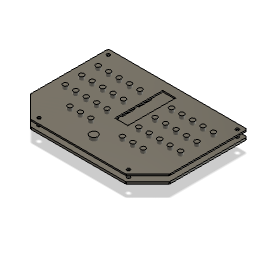
HandyPi_Keyboard (Autodesk Fusion 360 design; units mm, degrees)
Autodesk Fusion 360 part; units mm, degrees
(part 1 of 2)
sketch "basePCB" plane through (0, 0, 0) normal (0, 1, 0) x (1, 0, 0)
  line L0 (-37.295, 35.389) -> (-37.295, 28.289)
  circle A0 centre (-43.588, 31.486) radius 2.25
  line L1 (-37.295, 28.289) -> (-34.895, 28.289)
  line L2 (-0.936, -12.156) -> (-3.436, -12.156)
  line L3 (-28.672, 28.162) -> (-28.672, 35.262)
  line L4 (1.39, -12.156) -> (1.39, -16.756)
  line L5 (3.89, -12.156) -> (1.39, -12.156)
  line L6 (-0.936, -16.756) -> (-0.936, -12.156)
  line L7 (-3.436, -12.156) -> (-3.436, -16.756)
  line L8 (1.39, -16.756) -> (3.89, -16.756)
  line L9 (-3.436, -16.756) -> (-0.936, -16.756)
  line L10 (3.89, -16.756) -> (3.89, -12.156)
  line L11 (-34.895, 35.389) -> (-37.295, 35.389)
  line L12 (-31.072, 28.162) -> (-28.672, 28.162)
  line L13 (-28.672, 35.262) -> (-31.072, 35.262)
  line L14 (-31.072, 35.262) -> (-31.072, 28.162)
  line L15 (-34.895, 28.289) -> (-34.895, 35.389)
  line L16 (-15.998, -11.806) -> (-15.998, -11.556)
  line L17 (-8.124, 25.528) -> (-8.374, 25.528)
  line L18 (31.5, 25.528) -> (31.25, 25.528)
  line L19 (23.626, -11.556) -> (23.376, -11.556)
  line L20 (31.572, 3.582) -> (31.572, 3.832)
  line L21 (31.5, 25.278) -> (31.5, 16.278)
  line L22 (8.252, -11.806) -> (8.252, -11.556)
  line L23 (-8.124, -11.806) -> (-8.124, -11.556)
  line L24 (31.5, -11.806) -> (31.5, -20.806)
  line L25 (23.626, 16.028) -> (23.626, 16.278)
  line L26 (-23.498, 25.528) -> (-23.248, 25.528)
  line L27 (16.126, 25.528) -> (16.376, 25.528)
  line L28 (-8.374, -8.76) -> (-8.124, -8.76)
  line L29 (-15.624, 0.49) -> (-15.624, 0.74)
  line L30 (23.376, -21.056) -> (23.626, -21.056)
  line L31 (-15.624, 16.028) -> (-15.624, 16.278)
  line L32 (-8.124, 16.028) -> (-8.124, 16.278)
  line L33 (15.752, -11.556) -> (15.502, -11.556)
  line L34 (8.252, 13.082) -> (8.502, 13.082)
  line L35 (24.25, 0.74) -> (31.25, 0.74)
  line L36 (15.752, 25.278) -> (15.752, 25.528)
  line L37 (-15.998, -8.76) -> (-15.998, -8.51)
  line L38 (-15.624, 16.278) -> (-15.624, 25.278)
  line L39 (24, 16.028) -> (24, 16.278)
  line L40 (8.252, 25.528) -> (8.502, 25.528)
  line L41 (15.752, -8.76) -> (15.752, -8.51)
  line L42 (31.5, 0.49) -> (31.5, -8.51)
  line L43 (8.252, 0.49) -> (8.252, 0.74)
  line L44 (16.126, -8.51) -> (16.126, 0.49)
  line L45 (15.752, -11.806) -> (15.752, -20.806)
  line L46 (8.502, 13.082) -> (15.502, 13.082)
  line L47 (23.626, -21.056) -> (23.626, -20.806)
  line L48 (15.752, 13.082) -> (15.502, 13.082)
  line L49 (16.376, -21.056) -> (16.126, -21.056)
  line L50 (16.126, 0.49) -> (16.126, 0.74)
  line L51 (31.874, -8.51) -> (31.874, 0.49)
  line L52 (23.626, 0.49) -> (23.626, -8.51)
  line L53 (-15.624, -11.556) -> (-15.374, -11.556)
  line L54 (16.376, 25.528) -> (23.376, 25.528)
  line L55 (31.5, 0.49) -> (31.5, 0.74)
  line L56 (31.5, -8.76) -> (31.5, -8.51)
  line L57 (31.874, 25.278) -> (31.874, 25.528)
  line L58 (-16.248, -8.76) -> (-15.998, -8.76)
  line L59 (24, -11.556) -> (24.25, -11.556)
  line L60 (8.502, 3.582) -> (8.252, 3.582)
  line L61 (31.5, -11.556) -> (31.25, -11.556)
  line L62 (39.374, -8.76) -> (39.374, -8.51)
  line L63 (31.322, 3.582) -> (24.322, 3.582)
  line L64 (16.126, -8.76) -> (16.126, -8.51)
  line L65 (-23.498, -8.51) -> (-23.498, 0.49)
  line L66 (16.126, 12.832) -> (16.126, 13.082)
  line L67 (24, 16.278) -> (24, 25.278)
  line L68 (15.502, -8.76) -> (15.752, -8.76)
  line L69 (24.25, -21.056) -> (24, -21.056)
  line L70 (23.626, 12.832) -> (23.626, 13.082)
  line L71 (-8.374, -21.056) -> (-8.124, -21.056)
  line L72 (-8.374, 16.028) -> (-15.374, 16.028)
  line L73 (24.25, 16.028) -> (24, 16.028)
  line L74 (16.126, -11.806) -> (16.126, -11.556)
  line L75 (-15.624, -20.806) -> (-15.624, -11.806)
  line L76 (15.752, -11.806) -> (15.752, -11.556)
  line L77 (-15.998, 0.74) -> (-16.248, 0.74)
  line L78 (24.322, 13.082) -> (31.322, 13.082)
  line L79 (-15.998, -11.806) -> (-15.998, -20.806)
  line L80 (31.322, 3.582) -> (31.572, 3.582)
  line L81 (16.126, 16.028) -> (16.126, 16.278)
  line L82 (39.124, -8.76) -> (39.374, -8.76)
  line L83 (-8.124, -21.056) -> (-8.124, -20.806)
  line L84 (23.626, 25.278) -> (23.626, 25.528)
  line L85 (23.626, 13.082) -> (23.376, 13.082)
  line L86 (-15.374, 0.74) -> (-8.374, 0.74)
  line L87 (8.502, -8.76) -> (8.252, -8.76)
  line L88 (39.124, 16.028) -> (39.374, 16.028)
  line L89 (-8.124, -11.556) -> (-8.374, -11.556)
  line L90 (31.572, 13.082) -> (31.322, 13.082)
  line L91 (31.5, 16.028) -> (31.5, 16.278)
  line L92 (-16.248, -21.056) -> (-15.998, -21.056)
  line L93 (-15.624, 25.278) -> (-15.624, 25.528)
  line L94 (32.196, 3.582) -> (31.946, 3.582)
  line L95 (39.374, 25.528) -> (39.124, 25.528)
  line L96 (8.252, -11.556) -> (8.502, -11.556)
  line L97 (16.376, 13.082) -> (23.376, 13.082)
  line L98 (31.5, -11.806) -> (31.5, -11.556)
  line L99 (8.502, 16.028) -> (8.252, 16.028)
  line L100 (15.502, 3.582) -> (15.752, 3.582)
  line L101 (24.072, 12.832) -> (24.072, 13.082)
  line L102 (-23.498, 25.278) -> (-23.498, 25.528)
  line L103 (8.252, 25.278) -> (8.252, 25.528)
  line L104 (-15.374, -21.056) -> (-15.624, -21.056)
  line L105 (15.502, 3.582) -> (8.502, 3.582)
  line L106 (-23.498, 0.74) -> (-23.248, 0.74)
  line L107 (8.502, -21.056) -> (8.252, -21.056)
  line L108 (16.126, -21.056) -> (16.126, -20.806)
  line L109 (31.25, -21.056) -> (31.5, -21.056)
  line L110 (8.502, 0.74) -> (15.502, 0.74)
  line L111 (39.446, 3.582) -> (39.446, 3.832)
  line L112 (39.196, 3.582) -> (39.446, 3.582)
  line L113 (-23.248, 0.74) -> (-16.248, 0.74)
  line L114 (15.752, 3.582) -> (15.752, 3.832)
  line L115 (15.502, -8.76) -> (8.502, -8.76)
  line L116 (39.446, 12.832) -> (39.446, 13.082)
  line L117 (-15.624, -11.806) -> (-15.624, -11.556)
  line L118 (39.374, 25.278) -> (39.374, 25.528)
  line L119 (-15.374, -11.556) -> (-8.374, -11.556)
  line L120 (-15.998, -21.056) -> (-15.998, -20.806)
  line L121 (16.376, -8.76) -> (16.126, -8.76)
  line L122 (-15.624, 25.528) -> (-15.374, 25.528)
  line L123 (31.5, 25.278) -> (31.5, 25.528)
  line L124 (15.752, 12.832) -> (15.752, 3.832)
  line L125 (16.376, 0.74) -> (23.376, 0.74)
  line L126 (-16.248, -21.056) -> (-23.248, -21.056)
  line L127 (16.376, 3.582) -> (16.126, 3.582)
  line L128 (23.376, 16.028) -> (16.376, 16.028)
  line L129 (-23.248, -8.76) -> (-23.498, -8.76)
  line L130 (16.376, -11.556) -> (23.376, -11.556)
  line L131 (24, 0.74) -> (24.25, 0.74)
  line L132 (-23.498, -8.76) -> (-23.498, -8.51)
  line L133 (-23.498, -11.556) -> (-23.248, -11.556)
  line L134 (23.376, -8.76) -> (23.626, -8.76)
  line L135 (32.124, 25.528) -> (39.124, 25.528)
  line L136 (31.874, 25.528) -> (32.124, 25.528)
  line L137 (8.252, -21.056) -> (8.252, -20.806)
  line L138 (16.126, 13.082) -> (16.376, 13.082)
  line L139 (32.124, -8.76) -> (31.874, -8.76)
  line L140 (39.124, 16.028) -> (32.124, 16.028)
  line L141 (39.374, 16.028) -> (39.374, 16.278)
  line L142 (24, 0.49) -> (24, 0.74)
  line L143 (23.626, 12.832) -> (23.626, 3.832)
  line L144 (-15.998, 0.49) -> (-15.998, 0.74)
  line L145 (-16.248, -8.76) -> (-23.248, -8.76)
  line L146 (31.25, 16.028) -> (24.25, 16.028)
  line L147 (31.946, 3.582) -> (31.946, 3.832)
  line L148 (31.874, 16.278) -> (31.874, 25.278)
  line L149 (31.25, 16.028) -> (31.5, 16.028)
  line L150 (39.196, 3.582) -> (32.196, 3.582)
  line L151 (16.376, 16.028) -> (16.126, 16.028)
  line L152 (-8.374, -8.76) -> (-15.374, -8.76)
  line L153 (31.25, -8.76) -> (31.5, -8.76)
  line L154 (16.126, 0.74) -> (16.376, 0.74)
  line L155 (8.252, 3.582) -> (8.252, 3.832)
  line L156 (24.072, 3.582) -> (24.072, 3.832)
  line L157 (23.376, 3.582) -> (23.626, 3.582)
  line L158 (16.126, 3.832) -> (16.126, 12.832)
  line L159 (8.252, 16.028) -> (8.252, 16.278)
  line L160 (15.752, -21.056) -> (15.752, -20.806)
  line L161 (8.252, 16.278) -> (8.252, 25.278)
  line L162 (31.946, 3.832) -> (31.946, 12.832)
  line L163 (23.626, 0.74) -> (23.376, 0.74)
  line L164 (24.072, 13.082) -> (24.322, 13.082)
  line L165 (-15.624, -21.056) -> (-15.624, -20.806)
  line L166 (24.322, 3.582) -> (24.072, 3.582)
  line L167 (31.874, 16.028) -> (31.874, 16.278)
  line L168 (39.446, 13.082) -> (39.196, 13.082)
  line L169 (-8.374, 16.028) -> (-8.124, 16.028)
  line L170 (-8.124, 0.74) -> (-8.374, 0.74)
  line L171 (24, -11.806) -> (24, -11.556)
  line L172 (-15.374, 25.528) -> (-8.374, 25.528)
  line L173 (-8.124, -11.806) -> (-8.124, -20.806)
  line L174 (31.946, 12.832) -> (31.946, 13.082)
  line L175 (16.126, 25.278) -> (16.126, 25.528)
  line L176 (23.626, -8.76) -> (23.626, -8.51)
  line L177 (23.376, -8.76) -> (16.376, -8.76)
  line L178 (-8.124, -8.76) -> (-8.124, -8.51)
  line L179 (-15.374, -8.76) -> (-15.624, -8.76)
  line L180 (8.252, 0.74) -> (8.502, 0.74)
  line L181 (16.126, 3.582) -> (16.126, 3.832)
  line L182 (39.124, -8.76) -> (32.124, -8.76)
  line L183 (15.752, 0.49) -> (15.752, -8.51)
  line L184 (-15.374, 16.028) -> (-15.624, 16.028)
  line L185 (-15.998, 25.278) -> (-15.998, 25.528)
  line L186 (16.126, -20.806) -> (16.126, -11.806)
  line L187 (8.252, -8.76) -> (8.252, -8.51)
  line L188 (15.752, 16.028) -> (15.752, 16.278)
  line L189 (15.752, 0.74) -> (15.502, 0.74)
  line L190 (23.626, 25.528) -> (23.376, 25.528)
  line L191 (8.252, -20.806) -> (8.252, -11.806)
  line L192 (15.502, 16.028) -> (8.502, 16.028)
  line L193 (-15.624, -8.51) -> (-15.624, 0.49)
  line L194 (-23.248, -21.056) -> (-23.498, -21.056)
  line L195 (31.572, 12.832) -> (31.572, 13.082)
  line L196 (31.25, -8.76) -> (24.25, -8.76)
  line L197 (15.752, 0.49) -> (15.752, 0.74)
  line L198 (39.374, 0.49) -> (39.374, -8.51)
  line L199 (32.196, 13.082) -> (39.196, 13.082)
  line L200 (-23.498, 0.49) -> (-23.498, 0.74)
  line L201 (32.124, 0.74) -> (39.124, 0.74)
  line L202 (8.502, -11.556) -> (15.502, -11.556)
  line L203 (31.5, -21.056) -> (31.5, -20.806)
  line L204 (16.126, 16.278) -> (16.126, 25.278)
  line L205 (-15.998, -11.556) -> (-16.248, -11.556)
  line L206 (15.502, 16.028) -> (15.752, 16.028)
  line L207 (8.252, -8.51) -> (8.252, 0.49)
  line L208 (-8.124, 25.278) -> (-8.124, 16.278)
  line L209 (24, -21.056) -> (24, -20.806)
  line L210 (-23.498, -20.806) -> (-23.498, -11.806)
  line L211 (-8.124, 25.278) -> (-8.124, 25.528)
  line L212 (23.626, -11.806) -> (23.626, -11.556)
  line L213 (-15.998, 0.49) -> (-15.998, -8.51)
  line L214 (24, -8.51) -> (24, 0.49)
  line L215 (-8.124, 0.49) -> (-8.124, 0.74)
  line L216 (23.376, -21.056) -> (16.376, -21.056)
  line L217 (24, -20.806) -> (24, -11.806)
  line L218 (31.25, -21.056) -> (24.25, -21.056)
  line L219 (31.572, 12.832) -> (31.572, 3.832)
  line L220 (31.874, -8.76) -> (31.874, -8.51)
  line L221 (24.072, 3.832) -> (24.072, 12.832)
  line L222 (15.502, -21.056) -> (15.752, -21.056)
  line L223 (23.626, 3.582) -> (23.626, 3.832)
  line L224 (-8.374, -21.056) -> (-15.374, -21.056)
  line L225 (23.626, 0.49) -> (23.626, 0.74)
  line L226 (-23.248, -11.556) -> (-16.248, -11.556)
  line L227 (-15.624, -8.76) -> (-15.624, -8.51)
  line L228 (15.502, -21.056) -> (8.502, -21.056)
  line L229 (15.752, 25.278) -> (15.752, 16.278)
  line L230 (24.25, -11.556) -> (31.25, -11.556)
  line L231 (8.252, 3.832) -> (8.252, 12.832)
  line L232 (23.376, 3.582) -> (16.376, 3.582)
  line L233 (23.626, 25.278) -> (23.626, 16.278)
  line L234 (31.946, 13.082) -> (32.196, 13.082)
  line L235 (23.626, -11.806) -> (23.626, -20.806)
  line L236 (24, 25.528) -> (24.25, 25.528)
  line L237 (15.752, 12.832) -> (15.752, 13.082)
  line L238 (15.752, 25.528) -> (15.502, 25.528)
  line L239 (8.502, 25.528) -> (15.502, 25.528)
  line L240 (-23.498, -21.056) -> (-23.498, -20.806)
  line L241 (39.374, 25.278) -> (39.374, 16.278)
  line L242 (32.124, 16.028) -> (31.874, 16.028)
  line L243 (24, -8.76) -> (24, -8.51)
  line L244 (23.376, 16.028) -> (23.626, 16.028)
  line L245 (39.446, 12.832) -> (39.446, 3.832)
  line L246 (-15.998, 25.528) -> (-16.248, 25.528)
  line L247 (16.126, -11.556) -> (16.376, -11.556)
  line L248 (31.5, 0.74) -> (31.25, 0.74)
  line L249 (-8.124, 0.49) -> (-8.124, -8.51)
  line L250 (24.25, 25.528) -> (31.25, 25.528)
  line L251 (24.25, -8.76) -> (24, -8.76)
  line L252 (-15.624, 0.74) -> (-15.374, 0.74)
  line L253 (24, 25.278) -> (24, 25.528)
  line L254 (-23.498, -11.806) -> (-23.498, -11.556)
  line L255 (8.252, 12.832) -> (8.252, 13.082)
  line L256 (-31.746, 3.582) -> (-31.746, 3.832)
  line L257 (-47.12, 3.582) -> (-47.12, 3.832)
  line L258 (44.166, 32.996) -> (44.166, 36.096)
  line L259 (-39.87, -8.76) -> (-46.87, -8.76)
  line L260 (-23.872, 25.278) -> (-23.872, 16.278)
  line L261 (-39.246, 3.582) -> (-39.246, 3.832)
  line L262 (-38.996, -8.76) -> (-39.246, -8.76)
  line L263 (-31.746, 0.74) -> (-31.996, 0.74)
  line L264 (-39.87, 3.582) -> (-46.87, 3.582)
  line L265 (16.322, 32.03) -> (28.582, 32.03)
  line L266 (-47.12, 16.028) -> (-47.12, 16.278)
  line L267 (44.166, 36.096) -> (38.066, 36.096)
  line L268 (-31.372, 3.582) -> (-31.372, 3.832)
  line L269 (47.124, 28.22) -> (47.124, 31.22)
  line L270 (-23.872, 25.528) -> (-24.122, 25.528)
  line L271 (-24.122, 16.028) -> (-31.122, 16.028)
  line L272 (-23.872, 0.49) -> (-23.872, 0.74)
  line L273 (-31.372, -11.556) -> (-31.122, -11.556)
  line L274 (-31.746, 12.832) -> (-31.746, 13.082)
  line L275 (-23.872, -11.556) -> (-24.122, -11.556)
  line L276 (-31.372, 13.082) -> (-31.122, 13.082)
  line L277 (-24.122, 3.582) -> (-23.872, 3.582)
  line L278 (-39.62, -8.76) -> (-39.62, -8.51)
  line L279 (-47.12, 25.528) -> (-46.87, 25.528)
  line L280 (-46.87, 25.528) -> (-39.87, 25.528)
  line L281 (-24.122, -8.76) -> (-23.872, -8.76)
  line L282 (-39.246, 16.028) -> (-39.246, 16.278)
  line L283 (-47.12, 0.49) -> (-47.12, 0.74)
  line L284 (-46.87, 3.582) -> (-47.12, 3.582)
  line L285 (-31.746, 0.49) -> (-31.746, 0.74)
  line L286 (-31.372, -21.056) -> (-31.372, -20.806)
  line L287 (-31.122, 25.528) -> (-24.122, 25.528)
  line L288 (-31.746, 16.028) -> (-31.746, 16.278)
  line L289 (-16.248, 16.028) -> (-23.248, 16.028)
  line L290 (-39.62, 25.278) -> (-39.62, 25.528)
  line L291 (-31.746, 13.082) -> (-31.996, 13.082)
  line L292 (-23.872, 0.74) -> (-24.122, 0.74)
  line L293 (-23.872, -8.76) -> (-23.872, -8.51)
  line L294 (-47.12, 3.832) -> (-47.12, 12.832)
  line L295 (38.066, 36.096) -> (38.066, 32.996)
  line L296 (-31.122, 0.74) -> (-24.122, 0.74)
  line L297 (16.068, 28.22) -> (28.328, 28.22)
  line L298 (-24.122, -21.056) -> (-23.872, -21.056)
  line L299 (34.864, 31.22) -> (34.864, 28.22)
  line L300 (-23.248, 16.028) -> (-23.498, 16.028)
  line L301 (-31.996, -8.76) -> (-38.996, -8.76)
  line L302 (-31.996, 16.028) -> (-31.746, 16.028)
  line L303 (-39.246, 25.528) -> (-38.996, 25.528)
  line L304 (-39.87, 3.582) -> (-39.62, 3.582)
  line L305 (28.328, 28.22) -> (28.328, 31.22)
  line L306 (-24.122, -21.056) -> (-31.122, -21.056)
  line L307 (-31.746, 25.278) -> (-31.746, 25.528)
  line L308 (-39.246, 0.49) -> (-39.246, 0.74)
  line L309 (-38.996, 13.082) -> (-31.996, 13.082)
  line L310 (-47.12, -8.51) -> (-47.12, 0.49)
  line L311 (-23.872, -11.806) -> (-23.872, -11.556)
  line L312 (-39.62, 13.082) -> (-39.87, 13.082)
  line L313 (-31.996, -8.76) -> (-31.746, -8.76)
  line L314 (-31.372, 0.49) -> (-31.372, 0.74)
  line L315 (-31.372, 25.528) -> (-31.122, 25.528)
  line L316 (-39.87, 16.028) -> (-39.62, 16.028)
  line L317 (16.322, 35.03) -> (16.322, 32.03)
  line L318 (-31.122, -21.056) -> (-31.372, -21.056)
  line L319 (-16.248, 16.028) -> (-15.998, 16.028)
  line L320 (-23.872, 12.832) -> (-23.872, 3.832)
  line L321 (-31.746, 25.528) -> (-31.996, 25.528)
  line L322 (28.582, 32.03) -> (28.582, 35.03)
  line L323 (-46.87, 13.082) -> (-39.87, 13.082)
  line L324 (-23.248, 25.528) -> (-16.248, 25.528)
  line L325 (-23.872, 3.582) -> (-23.872, 3.832)
  line L326 (-31.372, -8.51) -> (-31.372, 0.49)
  line L327 (-31.996, 16.028) -> (-38.996, 16.028)
  line L328 (-39.62, 12.832) -> (-39.62, 13.082)
  line L329 (-39.246, 3.832) -> (-39.246, 12.832)
  line L330 (-39.62, 3.582) -> (-39.62, 3.832)
  line L331 (-23.498, 16.278) -> (-23.498, 25.278)
  line L332 (-31.122, -8.76) -> (-31.372, -8.76)
  line L333 (-31.746, 25.278) -> (-31.746, 16.278)
  line L334 (-31.996, 3.582) -> (-31.746, 3.582)
  line L335 (-39.87, 16.028) -> (-46.87, 16.028)
  line L336 (-46.87, -8.76) -> (-47.12, -8.76)
  line L337 (38.066, 32.996) -> (44.166, 32.996)
  line L338 (-23.302, 28.22) -> (-11.042, 28.22)
  line L339 (-31.372, 0.74) -> (-31.122, 0.74)
  line L340 (-31.372, 25.278) -> (-31.372, 25.528)
  line L341 (-46.87, 0.74) -> (-39.87, 0.74)
  line L342 (-31.372, -11.806) -> (-31.372, -11.556)
  line L343 (-39.246, 0.74) -> (-38.996, 0.74)
  line L344 (-46.87, 16.028) -> (-47.12, 16.028)
  line L345 (-31.372, 16.028) -> (-31.372, 16.278)
  line L346 (-39.62, 0.49) -> (-39.62, -8.51)
  line L347 (-31.996, 3.582) -> (-38.996, 3.582)
  line L348 (-47.12, 16.278) -> (-47.12, 25.278)
  line L349 (-31.372, -8.76) -> (-31.372, -8.51)
  line L350 (28.328, 31.22) -> (16.068, 31.22)
  line L351 (-39.62, 16.028) -> (-39.62, 16.278)
  line L352 (-24.122, 3.582) -> (-31.122, 3.582)
  line L353 (-11.042, 28.22) -> (-11.042, 31.22)
  line L354 (-23.872, 0.49) -> (-23.872, -8.51)
  line L355 (-31.372, -20.806) -> (-31.372, -11.806)
  line L356 (-23.872, 12.832) -> (-23.872, 13.082)
  line L357 (-23.872, 25.278) -> (-23.872, 25.528)
  line L358 (34.864, 28.22) -> (47.124, 28.22)
  line L359 (-31.746, 0.49) -> (-31.746, -8.51)
  line L360 (-47.12, 0.74) -> (-46.87, 0.74)
  line L361 (-39.62, 0.49) -> (-39.62, 0.74)
  line L362 (-24.122, 16.028) -> (-23.872, 16.028)
  line L363 (-39.62, 12.832) -> (-39.62, 3.832)
  line L364 (-15.998, 16.028) -> (-15.998, 16.278)
  line L365 (-38.996, 3.582) -> (-39.246, 3.582)
  line L366 (-47.12, 25.278) -> (-47.12, 25.528)
  line L367 (-23.872, 13.082) -> (-24.122, 13.082)
  line L368 (-39.246, -8.76) -> (-39.246, -8.51)
  line L369 (47.124, 31.22) -> (34.864, 31.22)
  line L370 (-38.996, 16.028) -> (-39.246, 16.028)
  line L371 (-39.246, -8.51) -> (-39.246, 0.49)
  line L372 (-31.122, -11.556) -> (-24.122, -11.556)
  line L373 (-39.87, -8.76) -> (-39.62, -8.76)
  line L374 (28.582, 35.03) -> (16.322, 35.03)
  line L375 (-39.62, 25.278) -> (-39.62, 16.278)
  line L376 (-39.62, 25.528) -> (-39.87, 25.528)
  line L377 (-24.122, -8.76) -> (-31.122, -8.76)
  line L378 (-23.872, 16.028) -> (-23.872, 16.278)
  line L379 (-31.746, -8.76) -> (-31.746, -8.51)
  line L380 (-39.62, 0.74) -> (-39.87, 0.74)
  line L381 (-47.12, -8.76) -> (-47.12, -8.51)
  line L382 (-31.122, 16.028) -> (-31.372, 16.028)
  line L383 (-31.122, 3.582) -> (-31.372, 3.582)
  line L384 (-23.302, 31.22) -> (-23.302, 28.22)
  line L385 (16.068, 31.22) -> (16.068, 28.22)
  line L386 (-39.246, 12.832) -> (-39.246, 13.082)
  line L387 (-39.246, 13.082) -> (-38.996, 13.082)
  line L388 (-38.996, 25.528) -> (-31.996, 25.528)
  line L389 (-47.12, 13.082) -> (-46.87, 13.082)
  line L390 (-31.372, 3.832) -> (-31.372, 12.832)
  line L391 (-23.872, -21.056) -> (-23.872, -20.806)
  line L392 (-31.372, 16.278) -> (-31.372, 25.278)
  line L393 (-47.12, 12.832) -> (-47.12, 13.082)
  line L394 (-31.372, 12.832) -> (-31.372, 13.082)
  line L395 (-39.246, 16.278) -> (-39.246, 25.278)
  line L396 (-38.996, 0.74) -> (-31.996, 0.74)
  line L397 (-23.872, -11.806) -> (-23.872, -20.806)
  line L398 (-15.998, 25.278) -> (-15.998, 16.278)
  line L399 (-11.042, 31.22) -> (-23.302, 31.22)
  line L400 (-31.122, 13.082) -> (-24.122, 13.082)
  line L401 (-31.746, 12.832) -> (-31.746, 3.832)
  line L402 (-39.246, 25.278) -> (-39.246, 25.528)
  line L403 (-23.498, 16.028) -> (-23.498, 16.278)
  line L404 (46.998, 16.028) -> (39.998, 16.028)
  line L405 (4.99, 31.016) -> (-4.81, 31.016)
  line L406 (47.248, 16.028) -> (47.248, 16.278)
  line L407 (-15.998, 3.582) -> (-15.998, 3.832)
  line L408 (46.998, -8.76) -> (39.998, -8.76)
  line L409 (39.998, 3.582) -> (39.748, 3.582)
  line L410 (-11.958, 35.334) -> (-15.558, 35.334)
  line L411 (-23.248, 13.082) -> (-16.248, 13.082)
  line L412 (-8.124, 12.832) -> (-8.124, 13.082)
  line L413 (46.998, 16.028) -> (47.248, 16.028)
  line L414 (-8.124, 12.832) -> (-8.124, 3.832)
  line L415 (-19.07, 32.234) -> (-19.07, 35.334)
  line L416 (39.748, -8.51) -> (39.748, 0.49)
  line L417 (-8.124, 13.082) -> (-8.374, 13.082)
  line L418 (4.99, -5.084) -> (4.99, 31.016)
  line L419 (39.748, 16.278) -> (39.748, 25.278)
  line L420 (39.374, 0.49) -> (39.374, 0.74)
  line L421 (39.748, -8.76) -> (39.748, -8.51)
  line L422 (-51.208, 37.594) -> (51.154, 37.594)
  arc A1 (-51.208, 37.594) -> (-52.478, 36.324) centre (-51.208, 36.324) ccw
  line L423 (-15.624, 3.582) -> (-15.624, 3.832)
  line L424 (-4.81, 31.016) -> (-4.81, -5.084)
  line L425 (-16.248, 3.582) -> (-23.248, 3.582)
  line L426 (-15.374, 3.582) -> (-15.624, 3.582)
  line L427 (39.748, 12.832) -> (39.748, 13.082)
  line L428 (39.998, 16.028) -> (39.748, 16.028)
  circle A2 centre (48.614, -33.78) radius 2.45
  line L429 (46.998, 3.582) -> (39.998, 3.582)
  line L430 (51.154, -37.59) -> (-51.208, -37.59)
  line L431 (-8.374, 3.582) -> (-8.124, 3.582)
  circle A3 centre (-48.668, -33.78) radius 2.45
  line L432 (39.748, 3.582) -> (39.748, 3.832)
  line L433 (-15.998, 13.082) -> (-16.248, 13.082)
  line L434 (-23.498, 12.832) -> (-23.498, 13.082)
  line L435 (39.748, 13.082) -> (39.998, 13.082)
  line L436 (47.248, 25.528) -> (46.998, 25.528)
  line L437 (-15.374, 13.082) -> (-8.374, 13.082)
  line L438 (39.998, 13.082) -> (46.998, 13.082)
  line L439 (39.998, -8.76) -> (39.748, -8.76)
  arc A4 (52.424, 36.324) -> (51.154, 37.594) centre (51.154, 36.324) ccw
  line L440 (31.874, 0.74) -> (32.124, 0.74)
  line L441 (39.374, 0.74) -> (39.124, 0.74)
  line L442 (39.748, 25.278) -> (39.748, 25.528)
  line L443 (47.248, 0.74) -> (46.998, 0.74)
  line L444 (6.14, -11.688) -> (6.14, -6.088)
  line L445 (39.748, 3.832) -> (39.748, 12.832)
  line L446 (-5.76, -11.688) -> (6.14, -11.688)
  line L447 (39.748, 0.49) -> (39.748, 0.74)
  line L448 (-16.248, 3.582) -> (-15.998, 3.582)
  line L449 (39.998, 25.528) -> (46.998, 25.528)
  line L450 (-23.248, 3.582) -> (-23.498, 3.582)
  line L451 (-8.124, 3.582) -> (-8.124, 3.832)
  line L452 (-15.558, 35.334) -> (-15.558, 32.234)
  line L453 (-52.478, -36.32) -> (-52.478, 36.324)
  line L454 (6.14, -6.088) -> (-5.76, -6.088)
  arc A5 (-52.478, -36.32) -> (-51.208, -37.59) centre (-51.208, -36.32) ccw
  line L455 (-22.67, 32.234) -> (-19.07, 32.234)
  line L456 (-23.498, 3.582) -> (-23.498, 3.832)
  line L457 (-4.81, -5.084) -> (4.99, -5.084)
  line L458 (39.748, 16.028) -> (39.748, 16.278)
  line L459 (-8.374, 3.582) -> (-15.374, 3.582)
  line L460 (-15.624, 3.832) -> (-15.624, 12.832)
  line L461 (39.748, 25.528) -> (39.998, 25.528)
  line L462 (-19.07, 35.334) -> (-22.67, 35.334)
  arc A6 (51.154, -37.59) -> (52.424, -36.32) centre (51.154, -36.32) ccw
  line L463 (-11.958, 32.234) -> (-11.958, 35.334)
  line L464 (31.874, 0.49) -> (31.874, 0.74)
  circle A7 centre (48.614, 33.784) radius 2.45
  line L465 (-23.498, 13.082) -> (-23.248, 13.082)
  line L466 (46.998, 3.582) -> (47.248, 3.582)
  circle A8 centre (-48.668, 33.784) radius 2.45
  line L467 (47.248, -8.76) -> (47.248, -8.51)
  line L468 (39.748, 0.74) -> (39.998, 0.74)
  line L469 (-15.998, 12.832) -> (-15.998, 13.082)
  line L470 (47.248, 0.49) -> (47.248, 0.74)
  line L471 (-5.76, -6.088) -> (-5.76, -11.688)
  line L472 (47.248, 3.582) -> (47.248, 3.832)
  line L473 (47.248, 12.832) -> (47.248, 3.832)
  line L474 (46.998, -8.76) -> (47.248, -8.76)
  line L475 (-15.998, 12.832) -> (-15.998, 3.832)
  line L476 (47.248, 0.49) -> (47.248, -8.51)
  line L477 (47.248, 25.278) -> (47.248, 25.528)
  line L478 (-15.624, 12.832) -> (-15.624, 13.082)
  line L479 (-23.498, 3.832) -> (-23.498, 12.832)
  line L480 (-22.67, 35.334) -> (-22.67, 32.234)
  line L481 (-15.558, 32.234) -> (-11.958, 32.234)
  line L482 (47.248, 25.278) -> (47.248, 16.278)
  line L483 (47.248, 13.082) -> (46.998, 13.082)
  line L484 (52.424, 36.324) -> (52.424, -36.32)
  line L485 (39.998, 0.74) -> (46.998, 0.74)
  line L486 (-15.624, 13.082) -> (-15.374, 13.082)
  line L487 (47.248, 12.832) -> (47.248, 13.082)
  circle A9 centre (48.614, 33.784) radius 1.25
  circle A10 centre (-48.668, 33.784) radius 1.25
  circle A11 centre (-48.668, -33.78) radius 1.25
  circle A12 centre (48.614, -33.78) radius 1.25
  dimension "d114" = 2.5
  dimension "d115" = 2.5
  dimension "d116" = 2.5
  dimension "d117" = 2.5
  constraint concentric A7 A9
  constraint concentric A8 A10
  constraint concentric A3 A11
  constraint concentric A2 A12
  measures "d114" diameter of A9
  measures "d115" diameter of A10
  measures "d116" diameter of A11
  measures "d117" diameter of A12
sketch "keys" plane through (0, 0, 0) normal (0, 1, 0) x (1, 0, 0)
  line L0 (-39.6574, 25.528) -> (-47.1574, 25.528)
  line L1 (-47.1574, 25.528) -> (-47.1574, 16.028)
  line L2 (-47.1574, 16.028) -> (-39.6574, 16.028)
  line L3 (-39.6574, 16.028) -> (-39.6574, 25.528)
  line L4 (-39.6574, 25.528) -> (-47.1574, 16.028) construction
  line L5 (-47.1574, 25.528) -> (-39.6574, 16.028) construction
  circle A0 centre (-43.4074, 20.778) radius 1.75
  line L6 (-47.1574, 13.128) -> (-47.1574, 3.628)
  line L7 (-47.1574, 13.128) -> (-39.6574, 3.628) construction
  line L8 (-39.6574, 3.628) -> (-39.6574, 13.128)
  line L9 (-47.1574, 3.628) -> (-39.6574, 3.628)
  circle A1 centre (-43.4074, 8.378) radius 1.75
  line L10 (-39.6574, 13.128) -> (-47.1574, 13.128)
  line L11 (-39.6574, 13.128) -> (-47.1574, 3.628) construction
  line L12 (-47.1574, 0.728) -> (-39.6574, -8.772) construction
  line L13 (-39.6574, -8.772) -> (-39.6574, 0.728)
  line L14 (-39.6574, 0.728) -> (-47.1574, -8.772) construction
  line L15 (-47.1574, -8.772) -> (-39.6574, -8.772)
  circle A2 centre (-43.4074, -4.022) radius 1.75
  line L16 (-39.6574, 0.728) -> (-47.1574, 0.728)
  line L17 (-47.1574, 0.728) -> (-47.1574, -8.772)
  line L18 (-39.2574, -8.772) -> (-31.7574, -8.772)
  circle A3 centre (-35.5074, -4.022) radius 1.75
  line L19 (-39.2574, 0.728) -> (-31.7574, -8.772) construction
  line L20 (-31.7574, 3.628) -> (-31.7574, 13.128)
  line L21 (-31.7574, 0.728) -> (-39.2574, -8.772) construction
  line L22 (-31.7574, -8.772) -> (-31.7574, 0.728)
  line L23 (-39.2574, 0.728) -> (-39.2574, -8.772)
  line L24 (-31.7574, 13.128) -> (-39.2574, 3.628) construction
  line L25 (-39.2574, 3.628) -> (-31.7574, 3.628)
  line L26 (-39.2574, 13.128) -> (-31.7574, 3.628) construction
  line L27 (-31.7574, 13.128) -> (-39.2574, 13.128)
  line L28 (-39.2574, 25.528) -> (-31.7574, 16.028) construction
  line L29 (-31.7574, 25.528) -> (-39.2574, 25.528)
  circle A4 centre (-35.5074, 8.378) radius 1.75
  line L30 (-39.2574, 13.128) -> (-39.2574, 3.628)
  line L31 (-39.2574, 16.028) -> (-31.7574, 16.028)
  line L32 (-31.7574, 16.028) -> (-31.7574, 25.528)
  line L33 (-31.7574, 0.728) -> (-39.2574, 0.728)
  line L34 (-39.2574, 25.528) -> (-39.2574, 16.028)
  circle A5 centre (-35.5074, 20.778) radius 1.75
  line L35 (-31.7574, 25.528) -> (-39.2574, 16.028) construction
  line L36 (-15.9574, 0.728) -> (-23.4574, -8.772) construction
  line L37 (-23.8574, 0.728) -> (-31.3574, -8.772) construction
  line L38 (-31.3574, 0.728) -> (-23.8574, -8.772) construction
  circle A6 centre (-27.6074, -4.022) radius 1.75
  line L39 (-31.3574, 0.728) -> (-31.3574, -8.772)
  line L40 (-23.8574, -8.772) -> (-23.8574, 0.728)
  line L41 (-23.4574, 0.728) -> (-23.4574, -8.772)
  line L42 (-23.4574, 0.728) -> (-15.9574, -8.772) construction
  line L43 (-15.9574, -8.772) -> (-15.9574, 0.728)
  line L44 (-15.9574, 0.728) -> (-23.4574, 0.728)
  line L45 (-23.4574, 3.628) -> (-15.9574, 3.628)
  line L46 (-23.4574, 16.028) -> (-15.9574, 16.028)
  circle A7 centre (-19.7074, 20.778) radius 1.75
  circle A8 centre (-27.6074, 8.378) radius 1.75
  line L47 (-23.4574, 25.528) -> (-15.9574, 16.028) construction
  line L48 (-23.4574, 25.528) -> (-23.4574, 16.028)
  line L49 (-23.4574, -8.772) -> (-15.9574, -8.772)
  line L50 (-31.3574, 25.528) -> (-31.3574, 16.028)
  line L51 (-15.9574, 13.128) -> (-23.4574, 13.128)
  line L52 (-23.8574, 0.728) -> (-31.3574, 0.728)
  line L53 (-15.9574, 16.028) -> (-15.9574, 25.528)
  line L54 (-31.3574, -8.772) -> (-23.8574, -8.772)
  circle A9 centre (-19.7074, 8.378) radius 1.75
  line L55 (-15.9574, 25.528) -> (-23.4574, 25.528)
  line L56 (-15.9574, 13.128) -> (-23.4574, 3.628) construction
  line L57 (-23.8574, 13.128) -> (-31.3574, 3.628) construction
  line L58 (-23.4574, 13.128) -> (-15.9574, 3.628) construction
  line L59 (-31.3574, 13.128) -> (-23.8574, 3.628) construction
  circle A10 centre (-27.6074, 20.778) radius 1.75
  line L60 (-23.8574, 13.128) -> (-31.3574, 13.128)
  line L61 (-31.3574, 3.628) -> (-23.8574, 3.628)
  line L62 (-15.9574, 3.628) -> (-15.9574, 13.128)
  line L63 (-23.4574, 13.128) -> (-23.4574, 3.628)
  line L64 (-23.8574, 3.628) -> (-23.8574, 13.128)
  line L65 (-23.8574, 16.028) -> (-23.8574, 25.528)
  line L66 (-31.3574, 16.028) -> (-23.8574, 16.028)
  line L67 (-31.3574, 13.128) -> (-31.3574, 3.628)
  line L68 (-15.9574, 25.528) -> (-23.4574, 16.028) construction
  line L69 (-31.3574, 25.528) -> (-23.8574, 16.028) construction
  line L70 (-23.8574, 25.528) -> (-31.3574, 25.528)
  line L71 (-23.8574, 25.528) -> (-31.3574, 16.028) construction
  circle A11 centre (-19.7074, -4.022) radius 1.75
  line L72 (-8.1074, 13.128) -> (-15.6074, 13.128)
  line L73 (-15.6074, 3.628) -> (-8.1074, 3.628)
  line L74 (-8.1074, 25.528) -> (-15.6074, 16.028) construction
  line L75 (-15.6074, 13.128) -> (-15.6074, 3.628)
  line L76 (-8.1074, 16.028) -> (-8.1074, 25.528)
  circle A12 centre (-11.8574, 8.378) radius 1.75
  line L77 (-15.6074, 25.528) -> (-15.6074, 16.028)
  circle A13 centre (-11.8574, 20.778) radius 1.75
  line L78 (-8.1074, -8.772) -> (-8.1074, 0.728)
  circle A14 centre (-11.8574, -4.022) radius 1.75
  line L79 (-15.6074, 0.728) -> (-8.1074, -8.772) construction
  line L80 (-15.6074, 16.028) -> (-8.1074, 16.028)
  line L81 (-15.6074, 13.128) -> (-8.1074, 3.628) construction
  line L82 (-8.1074, 0.728) -> (-15.6074, 0.728)
  line L83 (-8.1074, 13.128) -> (-15.6074, 3.628) construction
  line L84 (-8.1074, 0.728) -> (-15.6074, -8.772) construction
  line L85 (-15.6074, 0.728) -> (-15.6074, -8.772)
  line L86 (-15.6074, -8.772) -> (-8.1074, -8.772)
  line L87 (-8.1074, 3.628) -> (-8.1074, 13.128)
  line L88 (-8.1074, 25.528) -> (-15.6074, 25.528)
  line L89 (-15.6074, 25.528) -> (-8.1074, 16.028) construction
  line L90 (-8.1074, -11.572) -> (-15.6074, -11.572)
  circle A15 centre (-27.6074, -16.322) radius 1.75
  line L91 (-23.8574, -11.572) -> (-31.3574, -21.072) construction
  line L92 (-15.6074, -11.572) -> (-8.1074, -21.072) construction
  line L93 (-8.1074, -21.072) -> (-8.1074, -11.572)
  line L94 (-8.1074, -11.572) -> (-15.6074, -21.072) construction
  circle A16 centre (-11.8574, -16.322) radius 1.75
  line L95 (-15.6074, -11.572) -> (-15.6074, -21.072)
  line L96 (-23.8574, -11.572) -> (-31.3574, -11.572)
  line L97 (-31.3574, -21.072) -> (-23.8574, -21.072)
  line L98 (-23.4574, -21.072) -> (-15.9574, -21.072)
  line L99 (-15.6074, -21.072) -> (-8.1074, -21.072)
  line L100 (-31.3574, -11.572) -> (-23.8574, -21.072) construction
  line L101 (-23.4574, -11.572) -> (-23.4574, -21.072)
  line L102 (-15.9574, -21.072) -> (-15.9574, -11.572)
  circle A17 centre (-19.7074, -16.322) radius 1.75
  line L103 (-23.4574, -11.572) -> (-15.9574, -21.072) construction
  line L104 (-31.3574, -11.572) -> (-31.3574, -21.072)
  line L105 (-15.9574, -11.572) -> (-23.4574, -11.572)
  line L106 (-15.9574, -11.572) -> (-23.4574, -21.072) construction
  line L107 (-23.8574, -21.072) -> (-23.8574, -11.572)
  line L108 (39.7926, 25.528) -> (39.7926, 16.028)
  line L109 (39.4426, 16.028) -> (39.4426, 25.528)
  line L110 (47.2926, 16.028) -> (47.2926, 25.528)
  line L111 (47.2926, 25.528) -> (39.7926, 25.528)
  line L112 (39.7926, 25.528) -> (47.2926, 16.028) construction
  line L113 (39.7926, 16.028) -> (47.2926, 16.028)
  circle A18 centre (43.5426, 20.778) radius 1.75
  line L114 (47.2926, 25.528) -> (39.7926, 16.028) construction
  line L115 (47.2926, 13.128) -> (39.7926, 13.128)
  line L116 (47.2926, 0.728) -> (39.7926, 0.728)
  line L117 (39.7926, 3.628) -> (47.2926, 3.628)
  line L118 (39.4426, 3.628) -> (39.4426, 13.128)
  line L119 (47.2926, 13.128) -> (39.7926, 3.628) construction
  line L120 (39.7926, 13.128) -> (47.2926, 3.628) construction
  circle A19 centre (43.5426, 8.378) radius 1.75
  line L121 (47.2926, 3.628) -> (47.2926, 13.128)
  line L122 (39.7926, 13.128) -> (39.7926, 3.628)
  line L123 (31.9426, 25.528) -> (31.9426, 16.028)
  line L124 (31.5426, 16.028) -> (31.5426, 25.528)
  circle A20 centre (35.6926, 20.778) radius 1.75
  line L125 (23.6426, 0.728) -> (16.1426, -8.772) construction
  line L126 (24.0426, 0.728) -> (24.0426, -8.772)
  line L127 (31.5426, -8.772) -> (31.5426, 0.728)
  line L128 (39.4426, -8.772) -> (39.4426, 0.728)
  line L129 (24.0426, 0.728) -> (31.5426, -8.772) construction
  line L130 (39.7926, 0.728) -> (47.2926, -8.772) construction
  circle A21 centre (43.5426, -4.022) radius 1.75
  circle A22 centre (19.8926, -4.022) radius 1.75
  line L131 (39.4426, 0.728) -> (31.9426, -8.772) construction
  line L132 (8.2426, 0.728) -> (15.7426, -8.772) construction
  line L133 (15.7426, -8.772) -> (15.7426, 0.728)
  line L134 (47.2926, 0.728) -> (39.7926, -8.772) construction
  line L135 (31.9426, 0.728) -> (31.9426, -8.772)
  line L136 (47.2926, -8.772) -> (47.2926, 0.728)
  line L137 (39.7926, 0.728) -> (39.7926, -8.772)
  line L138 (16.1426, 0.728) -> (16.1426, -8.772)
  line L139 (15.7426, 0.728) -> (8.2426, -8.772) construction
  circle A23 centre (11.9926, -4.022) radius 1.75
  line L140 (23.6426, -8.772) -> (23.6426, 0.728)
  circle A24 centre (35.6926, -4.022) radius 1.75
  circle A25 centre (27.7926, -4.022) radius 1.75
  line L141 (8.2426, 0.728) -> (8.2426, -8.772)
  line L142 (16.1426, 0.728) -> (23.6426, -8.772) construction
  line L143 (31.5426, 0.728) -> (24.0426, -8.772) construction
  line L144 (31.9426, 0.728) -> (39.4426, -8.772) construction
  circle A26 centre (35.6926, 8.378) radius 1.75
  line L145 (24.0426, 3.628) -> (31.5426, 3.628)
  line L146 (31.5426, 13.128) -> (24.0426, 13.128)
  line L147 (24.0426, 16.028) -> (31.5426, 16.028)
  line L148 (31.5426, 25.528) -> (24.0426, 16.028) construction
  line L149 (31.5426, 13.128) -> (24.0426, 3.628) construction
  line L150 (31.5426, 3.628) -> (31.5426, 13.128)
  line L151 (31.9426, 13.128) -> (31.9426, 3.628)
  line L152 (31.5426, 25.528) -> (24.0426, 25.528)
  line L153 (24.0426, 25.528) -> (31.5426, 16.028) construction
  circle A27 centre (27.7926, 20.778) radius 1.75
  line L154 (15.7426, -11.572) -> (8.2426, -21.072) construction
  circle A28 centre (27.7926, 8.378) radius 1.75
  line L155 (8.2426, -11.572) -> (15.7426, -21.072) construction
  line L156 (24.0426, 13.128) -> (31.5426, 3.628) construction
  line L157 (39.4426, 13.128) -> (31.9426, 13.128)
  line L158 (31.5426, 0.728) -> (24.0426, 0.728)
  line L159 (24.0426, -8.772) -> (31.5426, -8.772)
  line L160 (31.9426, 16.028) -> (39.4426, 16.028)
  line L161 (15.7426, -11.572) -> (8.2426, -11.572)
  line L162 (39.4426, 25.528) -> (31.9426, 16.028) construction
  circle A29 centre (11.9926, -16.322) radius 1.75
  line L163 (31.9426, 3.628) -> (39.4426, 3.628)
  line L164 (8.2426, -21.072) -> (15.7426, -21.072)
  line L165 (39.4426, 0.728) -> (31.9426, 0.728)
  line L166 (31.9426, 13.128) -> (39.4426, 3.628) construction
  line L167 (39.4426, 13.128) -> (31.9426, 3.628) construction
  line L168 (39.4426, 25.528) -> (31.9426, 25.528)
  line L169 (31.9426, 25.528) -> (39.4426, 16.028) construction
  line L170 (16.1426, 16.028) -> (23.6426, 16.028)
  line L171 (23.6426, 25.528) -> (16.1426, 25.528)
  line L172 (23.9926, -21.072) -> (31.4926, -21.072)
  line L173 (23.6426, 13.128) -> (16.1426, 13.128)
  line L174 (16.1426, 25.528) -> (16.1426, 16.028)
  line L175 (31.4926, -21.072) -> (31.4926, -11.572)
  line L176 (16.1426, -8.772) -> (23.6426, -8.772)
  line L177 (24.0426, 25.528) -> (24.0426, 16.028)
  circle A30 centre (19.8926, 8.378) radius 1.75
  line L178 (8.2426, -8.772) -> (15.7426, -8.772)
  line L179 (23.6426, 16.028) -> (23.6426, 25.528)
  line L180 (39.7926, -8.772) -> (47.2926, -8.772)
  line L181 (8.2426, -11.572) -> (8.2426, -21.072)
  line L182 (16.1426, 25.528) -> (23.6426, 16.028) construction
  circle A31 centre (19.8926, 20.778) radius 1.75
  line L183 (15.7426, 25.528) -> (8.2426, 16.028) construction
  line L184 (23.6426, 25.528) -> (16.1426, 16.028) construction
  line L185 (8.2426, 25.528) -> (15.7426, 16.028) construction
  line L186 (23.9926, -11.572) -> (23.9926, -21.072)
  line L187 (31.9426, -8.772) -> (39.4426, -8.772)
  line L188 (15.7426, 16.028) -> (15.7426, 25.528)
  line L189 (31.4926, -11.572) -> (23.9926, -21.072) construction
  line L190 (16.1426, -21.072) -> (23.6426, -21.072)
  line L191 (8.2426, 16.028) -> (15.7426, 16.028)
  line L192 (23.9926, -11.572) -> (31.4926, -21.072) construction
  circle A32 centre (11.9926, 20.778) radius 1.75
  line L193 (31.4926, -11.572) -> (23.9926, -11.572)
  circle A33 centre (27.7426, -16.322) radius 1.75
  line L194 (23.6426, -21.072) -> (23.6426, -11.572)
  line L195 (23.6426, -11.572) -> (16.1426, -11.572)
  line L196 (8.2426, 25.528) -> (8.2426, 16.028)
  line L197 (23.6426, -11.572) -> (16.1426, -21.072) construction
  line L198 (15.7426, 25.528) -> (8.2426, 25.528)
  line L199 (15.7426, 13.128) -> (8.2426, 13.128)
  line L200 (15.7426, 13.128) -> (8.2426, 3.628) construction
  line L201 (16.1426, -11.572) -> (23.6426, -21.072) construction
  line L202 (15.7426, 0.728) -> (8.2426, 0.728)
  line L203 (8.2426, 3.628) -> (15.7426, 3.628)
  line L204 (16.1426, -11.572) -> (16.1426, -21.072)
  line L205 (16.1426, 3.628) -> (23.6426, 3.628)
  line L206 (15.7426, -21.072) -> (15.7426, -11.572)
  line L207 (23.6426, 0.728) -> (16.1426, 0.728)
  circle A34 centre (19.8926, -16.322) radius 1.75
  line L208 (8.2426, 13.128) -> (15.7426, 3.628) construction
  circle A35 centre (11.9926, 8.378) radius 1.75
  line L209 (8.2426, 13.128) -> (8.2426, 3.628)
  line L210 (16.1426, 13.128) -> (16.1426, 3.628)
  line L211 (23.6426, 13.128) -> (16.1426, 3.628) construction
  line L212 (24.0426, 13.128) -> (24.0426, 3.628)
  line L213 (15.7426, 3.628) -> (15.7426, 13.128)
  line L214 (23.6426, 3.628) -> (23.6426, 13.128)
  line L215 (16.1426, 13.128) -> (23.6426, 3.628) construction
  line L216 (4.973, -30.9552) -> (-5.027, -30.9552)
  line L217 (-5.027, -30.9552) -> (-5.027, -20.9552)
  line L218 (-5.027, -20.9552) -> (4.973, -20.9552)
  line L219 (4.973, -20.9552) -> (4.973, -30.9552)
  line L220 (4.973, -30.9552) -> (-5.027, -20.9552) construction
  line L221 (-5.027, -30.9552) -> (4.973, -20.9552) construction
  circle A36 centre (-0.027, -25.9552) radius 3
  point P0 (-43.4074, 20.778)
  point P1 (-43.4074, 8.378)
  point P2 (-43.4074, -4.022)
  point P3 (-35.5074, -4.022)
  point P4 (-35.5074, 8.378)
  point P5 (-35.5074, 20.778)
  point P6 (-19.7074, -4.022)
  point P7 (-27.6074, -4.022)
  point P8 (-19.7074, 8.378)
  point P9 (-19.7074, 20.778)
  point P10 (-27.6074, 8.378)
  point P11 (-27.6074, 20.778)
  point P12 (-11.8574, 8.378)
  point P13 (-16.0074, 16.028)
  point P14 (-16.0074, 13.128)
  point P15 (-16.0074, 3.628)
  point P16 (-16.0074, 0.728)
  point P17 (-11.8574, 20.778)
  point P18 (-16.0074, 25.528)
  point P19 (-16.0074, -8.772)
  point P20 (-11.8574, -4.022)
  point P21 (-11.8574, -16.322)
  point P22 (-16.0074, -21.072)
  point P23 (-27.6074, -16.322)
  point P24 (-31.7574, -21.072)
  point P25 (-19.7074, -16.322)
  point P26 (-31.7574, -11.572)
  point P27 (-16.0074, -11.572)
  point P28 (43.5426, -4.022)
  point P29 (23.5926, -21.072)
  point P30 (19.8926, -4.022)
  point P31 (39.3926, 3.628)
  point P32 (39.3926, 25.528)
  point P33 (39.3926, -8.772)
  point P34 (11.9926, -4.022)
  point P35 (35.6926, 8.378)
  point P36 (19.8926, 8.378)
  point P37 (27.7926, 20.778)
  point P38 (19.8926, 20.778)
  point P39 (27.7926, -4.022)
  point P40 (11.9926, -16.322)
  point P41 (35.6926, 20.778)
  point P42 (27.7926, 8.378)
  point P43 (23.5926, -11.572)
  point P44 (7.8426, -21.072)
  point P45 (7.8426, -11.572)
  point P46 (19.8926, -16.322)
  point P47 (35.6926, -4.022)
  point P48 (11.9926, 8.378)
  point P49 (11.9926, 20.778)
  point P50 (43.5426, 8.378)
  point P51 (39.3926, 13.128)
  point P52 (43.5426, 20.778)
  point P53 (27.7426, -16.322)
  point P54 (39.3926, 0.728)
  point P55 (39.3926, 16.028)
  point P56 (-0.027, -25.9552)
  dimension "d3" = 7.5
  dimension "d4" = 9.5
  dimension "d5" = 3.5
  dimension "d6" = 7.5
  dimension "d7" = 9.5
  dimension "d8" = 3.5
  dimension "d9" = 7.5
  dimension "d10" = 9.5
  dimension "d11" = 3.5
  dimension "d12" = 7.5
  dimension "d13" = 9.5
  dimension "d14" = 3.5
  dimension "d15" = 7.5
  dimension "d16" = 9.5
  dimension "d17" = 3.5
  dimension "d18" = 7.5
  dimension "d19" = 9.5
  dimension "d20" = 3.5
  dimension "d21" = 7.5
  dimension "d22" = 9.5
  dimension "d23" = 3.5
  dimension "d24" = 7.5
  dimension "d25" = 9.5
  dimension "d26" = 3.5
  dimension "d27" = 7.5
  dimension "d28" = 9.5
  dimension "d29" = 3.5
  dimension "d30" = 7.5
  dimension "d31" = 9.5
  dimension "d32" = 3.5
  dimension "d33" = 7.5
  dimension "d34" = 9.5
  dimension "d35" = 3.5
  dimension "d36" = 7.5
  dimension "d37" = 9.5
  dimension "d38" = 3.5
  dimension "d39" = 7.5
  dimension "d40" = 9.5
  dimension "d41" = 3.5
  dimension "d42" = 7.5
  dimension "d43" = 9.5
  dimension "d44" = 3.5
  dimension "d45" = 7.5
  dimension "d46" = 9.5
  dimension "d47" = 3.5
  dimension "d48" = 7.5
  dimension "d49" = 9.5
  dimension "d50" = 3.5
  dimension "d51" = 7.5
  dimension "d52" = 9.5
  dimension "d53" = 3.5
  dimension "d54" = 7.5
  dimension "d55" = 9.5
  dimension "d56" = 3.5
  dimension "d57" = 7.5
  dimension "d58" = 9.5
  dimension "d59" = 3.5
  dimension "d60" = 7.5
  dimension "d61" = 9.5
  dimension "d62" = 3.5
  dimension "d63" = 7.5
  dimension "d64" = 9.5
  dimension "d65" = 3.5
  dimension "d66" = 7.5
  dimension "d67" = 9.5
  dimension "d68" = 3.5
  dimension "d69" = 7.5
  dimension "d70" = 9.5
  dimension "d71" = 3.5
  dimension "d72" = 7.5
  dimension "d73" = 9.5
  dimension "d74" = 3.5
  dimension "d75" = 7.5
  dimension "d76" = 9.5
  dimension "d77" = 3.5
  dimension "d78" = 7.5
  dimension "d79" = 9.5
  dimension "d80" = 3.5
  dimension "d81" = 7.5
  dimension "d82" = 9.5
  dimension "d83" = 3.5
  dimension "d84" = 7.5
  dimension "d85" = 9.5
  dimension "d86" = 3.5
  dimension "d87" = 7.5
  dimension "d88" = 9.5
  dimension "d89" = 3.5
  dimension "d90" = 7.5
  dimension "d91" = 9.5
  dimension "d92" = 3.5
  dimension "d93" = 7.5
  dimension "d94" = 9.5
  dimension "d95" = 3.5
  dimension "d96" = 7.5
  dimension "d97" = 9.5
  dimension "d98" = 3.5
  dimension "d99" = 7.5
  dimension "d100" = 9.5
  dimension "d101" = 3.5
  dimension "d102" = 7.5
  dimension "d103" = 9.5
  dimension "d104" = 3.5
  dimension "d105" = 7.5
  dimension "d106" = 9.5
  dimension "d107" = 3.5
  dimension "d108" = 7.5
  dimension "d109" = 9.5
  dimension "d110" = 3.5
  dimension "d111" = 10
  dimension "d112" = 10
  dimension "d113" = 6
  constraint horizontal L0
  constraint perpendicular L0 L1
  constraint parallel L0 L2
  constraint parallel L1 L3
  constraint coincident L4 P0
  constraint coincident L5 P0
  constraint coincident P0 A0.centre
  constraint horizontal L10
  constraint perpendicular L6 L10
  constraint parallel L9 L10
  constraint parallel L6 L8
  constraint coincident P1 L11
  constraint coincident P1 L7
  constraint coincident P1 A1.centre
  constraint horizontal L16
  constraint perpendicular L16 L17
  constraint parallel L15 L16
  constraint parallel L13 L17
  constraint coincident P2 L14
  constraint coincident P2 L12
  constraint coincident P2 A2.centre
  constraint horizontal L29
  constraint perpendicular L29 L34
  constraint parallel L29 L31
  constraint parallel L32 L34
  constraint coincident P5 L35
  constraint coincident P5 L28
  constraint coincident P5 A5.centre
  constraint horizontal L27
  constraint perpendicular L27 L30
  constraint parallel L25 L27
  constraint parallel L20 L30
  constraint coincident P4 L24
  constraint coincident P4 L26
  constraint coincident P4 A4.centre
  constraint horizontal L33
  constraint perpendicular L23 L33
  constraint parallel L18 L33
  constraint parallel L22 L23
  constraint coincident P3 L21
  constraint coincident P3 L19
  constraint coincident P3 A3.centre
  constraint horizontal L70
  constraint perpendicular L50 L70
  constraint parallel L66 L70
  constraint parallel L50 L65
  constraint coincident P11 L71
  constraint coincident P11 L69
  constraint coincident P11 A10.centre
  constraint horizontal L60
  constraint perpendicular L60 L67
  constraint parallel L60 L61
  constraint parallel L64 L67
  constraint coincident P10 L57
  constraint coincident P10 L59
  constraint coincident P10 A8.centre
  constraint horizontal L52
  constraint perpendicular L39 L52
  constraint parallel L52 L54
  constraint parallel L39 L40
  constraint coincident P7 L37
  constraint coincident P7 L38
  constraint coincident P7 A6.centre
  constraint horizontal L55
  constraint perpendicular L48 L55
  constraint parallel L46 L55
  constraint parallel L48 L53
  constraint coincident P9 L68
  constraint coincident P9 L47
  constraint coincident P9 A7.centre
  constraint horizontal L51
  constraint perpendicular L51 L63
  constraint parallel L45 L51
  constraint parallel L62 L63
  constraint coincident P8 L56
  constraint coincident P8 L58
  constraint coincident P8 A9.centre
  constraint horizontal L44
  constraint perpendicular L41 L44
  constraint parallel L44 L49
  constraint parallel L41 L43
  constraint coincident P6 L36
  constraint coincident P6 L42
  constraint coincident P6 A11.centre
  constraint horizontal L88
  constraint perpendicular L77 L88
  constraint parallel L80 L88
  constraint parallel L76 L77
  constraint coincident P17 L74
  constraint coincident P17 L89
  constraint coincident P17 A13.centre
  constraint horizontal L72
  constraint perpendicular L72 L75
  constraint parallel L72 L73
  constraint parallel L75 L87
  constraint coincident P12 L83
  constraint coincident P12 L81
  constraint coincident P12 A12.centre
  constraint horizontal L82
  constraint perpendicular L82 L85
  constraint parallel L82 L86
  constraint parallel L78 L85
  constraint coincident P20 L84
  constraint coincident P20 L79
  constraint coincident P20 A14.centre
  constraint horizontal L96
  constraint perpendicular L96 L104
  constraint parallel L96 L97
  constraint parallel L104 L107
  constraint coincident P23 L91
  constraint coincident P23 L100
  constraint coincident P23 A15.centre
  constraint horizontal L105
  constraint perpendicular L101 L105
  constraint parallel L98 L105
  constraint parallel L101 L102
  constraint coincident P25 L106
  constraint coincident P25 L103
  constraint coincident P25 A17.centre
  constraint horizontal L90
  constraint perpendicular L90 L95
  constraint parallel L90 L99
  constraint parallel L93 L95
  constraint coincident P21 L94
  constraint coincident P21 L92
  constraint coincident P21 A16.centre
  constraint horizontal L198
  constraint perpendicular L196 L198
  constraint parallel L191 L198
  constraint parallel L188 L196
  constraint coincident P49 L183
  constraint coincident P49 L185
  constraint coincident P49 A32.centre
  constraint horizontal L199
  constraint perpendicular L199 L209
  constraint parallel L199 L203
  constraint parallel L209 L213
  constraint coincident P48 L200
  constraint coincident P48 L208
  constraint coincident P48 A35.centre
  constraint horizontal L202
  constraint perpendicular L141 L202
  constraint parallel L178 L202
  constraint parallel L133 L141
  constraint coincident P34 L139
  constraint coincident P34 L132
  constraint coincident P34 A23.centre
  constraint horizontal L171
  constraint perpendicular L171 L174
  constraint parallel L170 L171
  constraint parallel L174 L179
  constraint coincident P38 L184
  constraint coincident P38 L182
  constraint coincident P38 A31.centre
  constraint horizontal L173
  constraint perpendicular L173 L210
  constraint parallel L173 L205
  constraint parallel L210 L214
  constraint coincident P36 L211
  constraint coincident P36 L215
  constraint coincident P36 A30.centre
  constraint horizontal L207
  constraint perpendicular L138 L207
  constraint parallel L176 L207
  constraint parallel L138 L140
  constraint coincident P30 L125
  constraint coincident P30 L142
  constraint coincident P30 A22.centre
  constraint horizontal L152
  constraint perpendicular L152 L177
  constraint parallel L147 L152
  constraint parallel L124 L177
  constraint coincident P37 L148
  constraint coincident P37 L153
  constraint coincident P37 A27.centre
  constraint horizontal L146
  constraint perpendicular L146 L212
  constraint parallel L145 L146
  constraint parallel L150 L212
  constraint coincident P42 L149
  constraint coincident P42 L156
  constraint coincident P42 A28.centre
  constraint horizontal L158
  constraint perpendicular L126 L158
  constraint parallel L158 L159
  constraint parallel L126 L127
  constraint coincident P39 L143
  constraint coincident P39 L129
  constraint coincident P39 A25.centre
  constraint horizontal L168
  constraint perpendicular L123 L168
  constraint parallel L160 L168
  constraint parallel L109 L123
  constraint coincident P41 L162
  constraint coincident P41 L169
  constraint coincident P41 A20.centre
  constraint horizontal L157
  constraint perpendicular L151 L157
  constraint parallel L157 L163